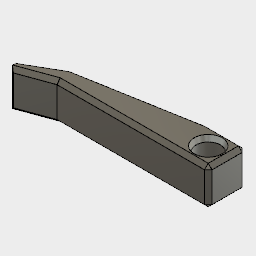
Toe (x4) (Autodesk Fusion 360 design; units mm, degrees)
Autodesk Fusion 360 part; units mm, degrees
sketch "Sketch3" plane through (0, 0, 0) normal (0, 1, 0) x (1, 0, 0)
  line L0 (0, 0) -> (-40, 0)
  line L1 (-40, 0) -> (-49.3969, -3.4202)
  line L2 (-40, 0) -> (-30, 0) construction
  line L3 (-49.3969, -3.4202) -> (-49.3969, -0.4202)
  line L4 (-49.3969, -0.4202) -> (-40.7346, 4.5763)
  line L5 (0, 0) -> (0, 10)
  line L6 (0, 10) -> (-10, 10)
  line L7 (-10, 10) -> (-40.7346, 4.5763)
  dimension "d3" = 40
  dimension "d4" = 160
  dimension "d5" = 10
  dimension "d6" = 3
  dimension "d7" = 10
  dimension "d8" = 10
  dimension "d9" = 10
  measures "d3" distance of L0.start L0.end
  measures "d4" angle of L1 L2
  measures "d5" distance of L0.end L1.end
  measures "d6" distance of L1.end L3.end
  measures "d7" distance of L3.end L4.end
  measures "d8" distance of L0.start L5.end
  measures "d9" distance of L5.end L6.end
extrude "Extrude1" add sketch "Sketch3" along normal blind 10
sketch "Sketch4" plane through (0, 10, 0) normal (0, 1, 0) x (-1, 0, 0)
  line L0 (0, 0) -> (0, -10)
  line L1 (0, -10) -> (10, -10)
  line L2 (10, -10) -> (40.7346, -4.5763)
  line L3 (40.7346, -4.5763) -> (49.3969, 0.4202)
  line L4 (49.3969, 0.4202) -> (49.3969, 3.4202)
  line L5 (49.3969, 3.4202) -> (40, 0)
  line L6 (40, 0) -> (0, 0)
  line L7 (0, 0) -> (10, 0)
  line L8 (0, -5) -> (5, -4.9937)
  circle A0 centre (5, -4.9937) radius 3.2
  dimension "d12" = 10
  dimension "d26" = 5
  dimension "d27" = 6.4
  measures "d12" distance of L0.start L7.end
  measures "d26" distance of L8.start L8.end
  measures "d27" diameter of A0
sketch "Sketch5" plane through (0, 0, 0) normal (0, -1, 0) x (1, 0, 0)
  line L0 (0, -10) -> (0, 0)
  line L1 (0, 0) -> (-40, 0)
  line L2 (-40, 0) -> (-49.3969, 3.4202)
  line L3 (-49.3969, 3.4202) -> (-49.3969, 0.4202)
  line L4 (-49.3969, 0.4202) -> (-40.7346, -4.5763)
  line L5 (-40.7346, -4.5763) -> (-10, -10)
  line L6 (-10, -10) -> (0, -10)
  line L7 (0, 0) -> (-10, 0)
  dimension "d13" = 10
  measures "d13" distance of L0.end L7.end
extrude "Extrude2" cut sketch "Sketch4" against normal blind 21 contours A0
chamfer "Chamfer1" distance 1 angle 45 8 edges at (0, 5, -10) (0, 5, 0) (-5, 10, -10) (0, 10, -5) (-20, 10, 0) (-20, 0, 0) (0, 0, -5) (-5, 0, -10)
chamfer "Chamfer2" distance 1 angle 45 1 edges at (-43.3247, 10, 1.2101)
chamfer "Chamfer3" distance 1 angle 45 1 edges at (-45.0658, 10, -2.078)
chamfer "Chamfer4" distance 1 angle 45 1 edges at (-28.2007, 0, -6.7881)
chamfer "Chamfer5" distance 1 angle 45 1 edges at (-26.7588, 10, -7.0426)
chamfer "Chamfer6" distance 1 angle 45 1 edges at (-40.7346, 5, -4.5763)
chamfer "Chamfer7" distance 1 angle 45 1 edges at (-49.3969, 4.5, 0.4202)
chamfer "Chamfer8" distance 1 angle 45 1 edges at (-45.9009, 0, -1.5963)
chamfer "Chamfer9" distance 1 angle 45 1 edges at (-43.3247, 0, 1.2101)
chamfer "Chamfer10" distance 1 angle 45 1 edges at (-49.3969, 5, 3.4202)
chamfer "Chamfer11" distance 0.5 angle 70 2 edges at (-2.0165, 0, -6.1508) (-2.0165, 10, -3.8365) measured on face at (-19.4177, 0, -4.8389) measured on face at (-19.4177, 10, -4.8389)
equation "d14 = ElephantFIT"
equation "ElephantFIT = 1 mm" comment "Chamfer by this amount"
equation "d16 = StyleFIT"
equation "d17 = StyleFIT"
equation "d18 = StyleFIT"
equation "d19 = StyleFIT"
equation "d20 = StyleFIT"
equation "d21 = StyleFIT"
equation "d22 = StyleFIT"
equation "d23 = StyleFIT"
equation "d24 = StyleFIT"
equation "StyleFIT = 1 mm"
equation "d26 = HolePosX"
equation "d27 = HoleSize"
equation "HoleSize = 6.4 mm"
equation "HolePosX = 5 mm"
equation "d32 = HoleFIT"
equation "d33 = HoleAngle"
equation "HoleFIT = 0.5 mm"
equation "HoleAngle = 70 deg"
